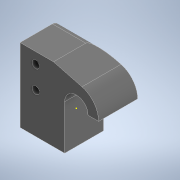
# Autodesk Inventor part: XAxisLimitSwitchMount
Saved by Autodesk Inventor 2022 (Build 260153000, 153)
## iProperties
Created: 2021-06-30
Part Number: XAxisLimitSwitchMount
Material: Generic
Document SubType Name: Modeling
Designer: BBL
Density: 1 g/cm^3
Appearance: Gray
Author: BBL
Autodesk Inventor part; units mm, degrees
ref_plane "YZ Plane" through (0, 0, 0) normal (1, 0, 0) x (0, 1, 0)
ref_plane "XZ Plane" through (0, 0, 0) normal (0, 1, 0) x (-1, 0, 0)
ref_plane "XY Plane" through (0, 0, 0) normal (0, 0, 1) x (1, 0, 0)
sketch "Sketch1" plane through (0, 0, 0) normal (0, 0, 1) x (1, 0, 0)
  arc A0 (5.25, 0) -> (-5.25, 0) centre (0, 0) ccw
  arc A1 (10, 0) -> (-3.960396, 9.182334) centre (0, 0) ccw
  line L0 (-5.25, -8.511022) -> (-5.25, -20)
  line L1 (-5.25, -20) -> (-25.25, -20)
  line L2 (-25.25, -20) -> (-25.25, 0)
  line L3 (5.25, 0) -> (10, 0)
  line L4 (-25.25, 0) -> (-3.960396, 9.182334)
  line L5 (-5.25, -8.511022) -> (-5.25, 0)
  line L6 (-25.25, 0) -> (-25.25, 13)
  line L7 (-25.25, 13) -> (-10.25, 13)
  line L8 (-10.25, 13) -> (2.706976, 9.628622)
  point P0 (1.153738, 9.933221)
  point P1 (2.518133, 9.677758)
  dimension "d0" = 10.5
  dimension "d1" = 20
  dimension "d3" = 20
  dimension "d5" = 20
  dimension "d6" = 0
  dimension "d7" = 20
  dimension "d14" = 13
  dimension "d18" = 15
  constraints: 18 end point, 5 point on circle, 4 perpendicular, 3 tangent, 3 vertical, 2 centre point, 2 coincident
  measures "d0" diameter of A0
  measures "d1" diameter of A1
  measures "d3" distance of L0.end L1.end
  measures "d5" vertical distance of point (0, 0) L0.end
  measures "d6" distance from line of point (0, 0) L3
  measures "d7" distance of L1.end L2.end
  measures "d14" distance of L2.end L6.end
  measures "d18" distance of L6.end L7.end
sketch "Sketch1 outline for Extrusion1" plane through (0, 0, 0) normal (0, 0, 1) x (1, 0, 0)
  arc A0 (10, 0) -> (2.518133, 9.677758) centre (0, 0) ccw
  line L0 (2.518133, 9.677758) -> (-10.25, 13)
  line L1 (-10.25, 13) -> (-25.25, 13)
  line L2 (-25.25, 13) -> (-25.25, -20)
  line L3 (-25.25, -20) -> (-5.25, -20)
  line L4 (-5.25, -20) -> (-5.25, 0)
  arc A1 (-5.25, 0) -> (5.25, 0) centre (0, 0) cw
  line L5 (5.25, 0) -> (10, 0)
extrude "Extrusion1" add sketch "Sketch1 outline for Extrusion1" along normal blind 17.5
sketch "Sketch3" plane through (0, 0, 17.5) normal (0, 0, 1) x (1, 0, 0)
  point P0 (0, 0)
sketch "Sketch4" plane through (0, 0, 0) normal (0, 0, -1) x (-1, 0, 0)
  arc A0 (-2.518133, 9.677758) -> (-10, 0) centre (0, 0) ccw
  line L0 (25.25, 13) -> (25.25, -20)
  arc A1 (-2.518133, 9.677758) -> (-10, 0) centre (0, 0) ccw
  line L1 (-5.25, 0) -> (-10, 0)
  arc A2 (5.25, 0) -> (-5.25, 0) centre (0, 0) ccw
  line L2 (5.25, -20) -> (5.25, 0)
  line L3 (25.25, -20) -> (5.25, -20)
  circle A3 centre (0, 0) radius 10
  line L4 (10, 11.228722) -> (10, -20)
  line L5 (25.25, -20) -> (5.25, -20)
  line L6 (10, 0) -> (25.25, 0)
  line L7 (25.25, 13) -> (25.25, -20)
  line L8 (10.25, 13) -> (25.25, 13)
  line L9 (-2.518133, 9.677758) -> (10.25, 13)
  point P0 (-1.153738, 9.933221)
  constraints: 4 end point, 3 point on line, 2 perpendicular, 1 coincident, 1 horizontal alignment, 2 other
extrude "Extrusion3" add sketch "Sketch4" along normal blind 10 contours L6 L0 L3 L4
fillet "Fillet1" radius 10 1 edges at (-17.625, 0, 0)
sketch "Sketch5" plane through (0, 0, 17.5) normal (0, 0, 1) x (1, 0, 0)
  line L0 (-25.25, 13) -> (-25.25, -20)
  line L1 (-25.25, -20) -> (-5.25, -20)
  line L2 (-5.25, -20) -> (-5.25, 0)
  arc A0 (5.25, 0) -> (-5.25, 0) centre (0, 0) ccw
  line L3 (5.25, 0) -> (10, 0)
  arc A1 (10, 0) -> (2.518133, 9.677758) centre (0, 0) ccw
  line L4 (2.518133, 9.677758) -> (-10.25, 13)
  line L5 (-10.25, 13) -> (-25.25, 13)
  circle A2 centre (-18.25, 8) radius 1.65
  circle A3 centre (-18.25, -2) radius 1.65
  dimension "d19" = 3.3
  dimension "d20" = 3.3
  dimension "d22" = 5
  dimension "d23" = 10
  dimension "d24" = 7
  dimension "d25" = 7
  constraints: 2 centre point
  measures "d19" diameter of A2
  measures "d20" diameter of A3
  measures "d22" distance from line of L5 A2.centre
  measures "d23" distance of A3.centre A2.centre
  measures "d24" distance from line of L0 A2.centre
  measures "d25" distance from line of L0 A3.centre
extrude "Extrusion4" cut sketch "Sketch5" against normal blind 15 contours A2 | A3
sketch "Sketch6" plane through (-25.25, -20, 17.5) normal (-1, 0, 0) x (0, 0, 1)
  line L0 (-7.5, 30.75) -> (-5, 30.75)
  line L1 (-5, 30.75) -> (-5, 25.25)
  line L2 (-5, 25.25) -> (-7.5, 25.25)
  line L3 (-7.5, 25.25) -> (-7.5, 30.75)
  line L4 (-7.5, 20.75) -> (-5, 20.75)
  line L5 (-5, 20.75) -> (-5, 15.25)
  line L6 (-5, 15.25) -> (-7.5, 15.25)
  line L7 (-7.5, 15.25) -> (-7.5, 20.75)
  line L8 (0, 19.65) -> (0, 16.35) projected
  line L9 (0, 29.65) -> (0, 26.35) projected
  point P0 (-17.5, 20)
  point P1 (-27.5, 16.35)
  point P2 (-27.5, 19.65)
  dimension "d28" = 5.5
  dimension "d29" = 5.5
  dimension "d30" = 2.5
  dimension "d31" = 2.5
  dimension "d32" = 0
  dimension "d33" = 5
  dimension "d34" = 3.3
  dimension "d35" = 1.1
  dimension "d36" = 1.1
  dimension "d37" = 1.1
  dimension "d38" = 1.1
  constraints: 16 end point, 4 parallel, 2 horizontal, 2 perpendicular
  measures "d28" distance between parallel lines of L6 L4
  measures "d29" distance between parallel lines of L0 L2
  measures "d30" distance of L5.end L6.end
  measures "d31" distance of L0.start L0.end
  measures "d32" distance between parallel lines of L1 L5
  measures "d33" distance between parallel lines of L8 L5
  measures "d34" distance of L8.start L8.end
  measures "d35" distance from line of L6 L8.end
  measures "d36" vertical distance of L8.start L4.end
  measures "d37" vertical distance of L9.end L1.end
  measures "d38" vertical distance of L9.start L0.end
extrude "Extrusion5" cut sketch "Sketch6" against normal blind 12
fillet "Fillet2" radius 3 1 edges at (-17.75, 13, 0)
equation "\"d7\" = d5"
equation "\"d29\" = d28"
equation "\"d31\" = d30"
equation "\"d35\" = -0.5 * d34 + 0.5 * d28"
equation "\"d37\" = d38"
body "Solid1"
